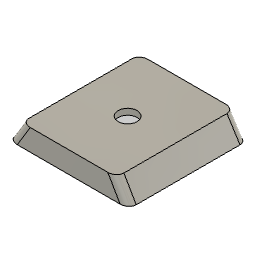
RP-10 QR Plate (Autodesk Fusion 360 design; units mm, degrees)
Autodesk Fusion 360 part; units mm, degrees
sketch "bottom" plane through (0, 0, 0) normal (0, 1, 0) x (1, 0, 0)
  line L0 (0, 0) -> (40, 0)
  line L1 (40, 0) -> (40, 39.5)
  line L2 (40, 39.5) -> (0, 39.5)
  line L3 (0, 39.5) -> (0, 0)
  dimension "d4" = 40
  dimension "d5" = 39.5
  constraint horizontal L0
  constraint vertical L1
  constraint horizontal L2
  constraint vertical L3
  constraint coincident L0.start L3.end
  measures "d4" distance of L0.start L0.end
  measures "d5" distance of L0.start L2.end
extrude "Extrude1" add sketch "bottom" along normal blind 7
draft "Draft1" angle 1 neutral plane through (0, 0, 0) pull (0, 1, 0) 1 faces at (13.3333, 2.3333, 0)
draft "Draft2" angle 31 neutral plane through (0, 0, 0) pull (0, 1, 0) 2 faces at (0, 2.3333, -13.2074) (40, 2.3333, -13.2074)
draft "Draft3" angle 1 neutral plane through (0, 0, 0) pull (0, 1, 0) 1 faces at (14.7353, 2.3333, -39.5)
shell "Shell1" thickness 2 removed faces 1 at (26.6667, 0, -13.1667)
sketch "top" plane through (0, 7, 0) normal (0, 1, 0) x (-1, 0, 0)
  line L0 (-4.206, -39.3778) -> (-4.206, -0.1222)
  line L1 (-4.206, -0.1222) -> (-35.794, -0.1222)
  line L2 (-35.794, -0.1222) -> (-35.794, -39.3778)
  line L3 (-35.794, -39.3778) -> (-4.206, -39.3778)
  line L4 (-20, -0.1222) -> (-20, -19.6222) construction
  circle A0 centre (-20, -19.6222) radius 3.175
  dimension "d23" = 19.5
  dimension "d25" = 6.35
  constraint midpoint L1 L4.start
  constraint perpendicular L1 L4
  constraint coincident L4.end A0.centre
  measures "d23" distance of L4.start L4.end
  measures "d25" diameter of A0
extrude "Extrude2" cut sketch "top" against normal blind 2 contours A0
fillet "Fillet1" radius 2.5 4 edges at (2.103, 3.5, -0.0611) (37.897, 3.5, -0.0611) (37.897, 3.5, -39.4389) (2.103, 3.5, -39.4389)
sketch "Sketch3" plane through (0, 0, 0) normal (0, 0.017452, 0.999848) x (1, 0, 0)
  line L0 (37.1096, 0) -> (32.9036, 7.0011)
  line L1 (32.9036, 7.0011) -> (7.0964, 7.0011)
  line L2 (7.0964, 7.0011) -> (2.8904, 0)
  line L3 (2.8904, 0) -> (37.1096, 0)
  line L4 (20, 7.0011) -> (20, 0) construction
  line L5 (4.9934, 3.5005) -> (35.0066, 3.5005) construction
  line L6 (4.9934, 1.7505) -> (35.0066, 1.7505) construction
  dimension "d31" = 1.75
  dimension "d32" = 3.5
  constraint midpoint L1 L4.start
  constraint midpoint L3 L4.end
  constraint midpoint L2 L5.start
  constraint midpoint L0 L5.end
extrude "Extrude3" [suppressed]
equation "PLATE_BASE_WIDTH = 40 mm"
equation "PLATE_BASE_HEIGHT = 39.5 mm"
equation "PLATE_HEIGHT = 7 mm"
equation "d4 = PLATE_BASE_WIDTH"
equation "d5 = PLATE_BASE_HEIGHT"
equation "d6 = PLATE_HEIGHT"
equation "DRAFT_SIDES = 31 deg"
equation "DRAFT_BACK = 1 deg"
equation "DRAFT_FRONT = 1 deg"
equation "d14 = DRAFT_FRONT"
equation "d16 = DRAFT_SIDES"
equation "d17 = DRAFT_SIDES"
equation "d18 = DRAFT_BACK"
equation "SHELL_THICKNESS = 2 mm"
equation "d21 = SHELL_THICKNESS"
equation "THREAD_OFFSET_FRONT = 20 mm"
equation "d23 = PLATE_BASE_HEIGHT - THREAD_OFFSET_FRONT"
equation "THREAD_HOLE_RAD = 0.25 in"
equation "d25 = THREAD_HOLE_RAD"
equation "d26 = -SHELL_THICKNESS"
equation "EDGE_FILLET = 2.5 mm"
equation "d30 = EDGE_FILLET"
equation "d31 = PLATE_HEIGHT / 4"
equation "d32 = PLATE_HEIGHT / 2"
named bodies: "RP-10 Quick Release Plate"
